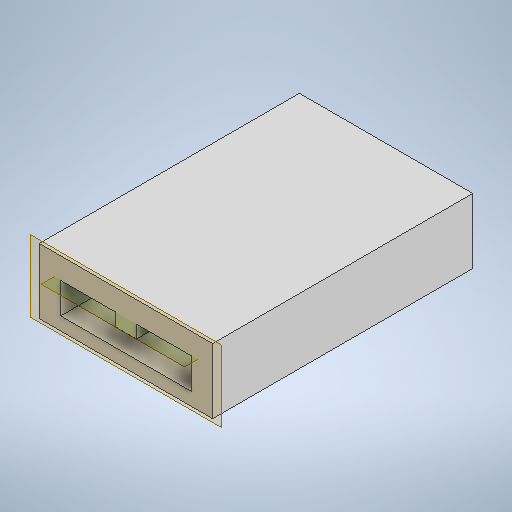
# Autodesk Inventor part: linia
Saved by Autodesk Inventor 2025.1 (Build 291241000, 241)
## iProperties
Created: 2024-11-25
Part Number: linia
Material: 一般
Document SubType Name: Modeling
Designer: dell
Density: 1 g/cm^3
Appearance: 既定
Author: dell
Autodesk Inventor part; units mm, degrees
ref_plane "YZ Plane" through (0, 0, 0) normal (1, 0, 0) x (0, 1, 0)
ref_plane "XZ Plane" through (0, 0, 0) normal (0, 1, 0) x (-1, 0, 0)
ref_plane "XY Plane" through (0, 0, 0) normal (0, 0, 1) x (1, 0, 0)
sketch "スケッチ1" plane through (0, 0, 0) normal (0, 1, 0) x (-1, 0, 0)
  line L0 (0, 0) -> (40, 0)
  line L1 (40, 0) -> (40, -60)
  line L2 (40, -60) -> (0, -60)
  line L3 (0, -60) -> (0, 0)
  dimension "d0" = 40
  dimension "d1" = 60
  constraints: 8 end point, 2 parallel, 1 horizontal, 1 perpendicular
  measures "d0" distance of L1.end L2.end
  measures "d1" distance of L0.end L1.end
extrude "押し出し1" add sketch "スケッチ1" along normal blind 15
ref_plane "作業平面1" through (-40, 0, 0) normal (0, 0, 1) x (1, 0, 0)
sketch "スケッチ2" plane through (-40, 0, 0) normal (0, 0, 1) x (1, 0, 0)
  line L0 (40, 15) -> (0, 15) projected
  line L1 (0, 0) -> (40, 0) projected
  line L2 (0, 0) -> (0, 15) projected
  line L3 (40, 0) -> (40, 15) projected
  line L4 (4.95, 3) -> (35.05, 3)
  line L5 (35.05, 3) -> (35.05, 10.1)
  line L6 (35.05, 10.1) -> (4.95, 10.1)
  line L7 (4.95, 10.1) -> (4.95, 3)
  point P0 (20, 10.1)
  dimension "d6" = 15
  dimension "d7" = 40
  dimension "d8" = 30.1
  dimension "d9" = 7.1
  dimension "d10" = 3
  constraints: 8 end point, 2 parallel, 1 horizontal, 1 midpoint, 1 perpendicular
  measures "d6" distance between parallel lines of L1 L0
  measures "d7" distance between parallel lines of L2 L3
  measures "d8" distance of L6.end L5.end
  measures "d9" distance of L5.end L4.end
  measures "d10" distance between parallel lines of L1 L4
extrude "押し出し2" cut sketch "スケッチ2" against normal through all contours L7 L6 L5 L4
ref_plane "作業平面2" through (-35.05, 10.1, -60) normal (0, -1, 0) x (1, 0, 0)
sketch "スケッチ3" plane through (-35.05, 10.1, -60) normal (0, -1, 0) x (1, 0, 0)
  line L0 (-4.95, 60) -> (35.05, 60) projected
  line L1 (12.6, 60) -> (17.5, 60)
  line L2 (17.5, 60) -> (17.5, 0)
  line L3 (17.5, 0) -> (12.6, 0)
  line L4 (12.6, 0) -> (12.6, 60)
  point P0 (15.05, 60)
  dimension "d15" = 60
  dimension "d16" = 4.9
  constraints: 8 end point, 2 parallel, 1 horizontal, 1 midpoint, 1 perpendicular, 1 point on line
  measures "d15" distance of L1.end L2.end
  measures "d16" distance between parallel lines of L2 L4
extrude "押し出し3" add sketch "スケッチ3" along normal blind 2.95
